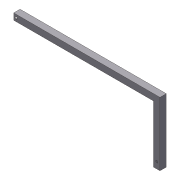
# Autodesk Inventor part: LoweringArm
Saved by Autodesk Inventor 2012 (Build 160160000, 160)
## iProperties
Created: 2012-02-26
Part Number: LoweringArm
Material: Aluminum-6061
Document SubType Name: Modeling
Designer: JesseK
Density: 2.71 g/cm^3
Mass: 259.596 g
Surface Area: 1210.8 cm^2
Volume: 95.7917 cm^3
Author: JesseK
Autodesk Inventor part; units mm, degrees
ref_plane "YZ Plane" through (0, 0, 0) normal (1, 0, 0) x (0, 1, 0)
ref_plane "XZ Plane" through (0, 0, 0) normal (0, 1, 0) x (-1, 0, 0)
ref_plane "XY Plane" through (0, 0, 0) normal (0, 0, 1) x (1, 0, 0)
sketch "Sketch1" plane through (0, 0, 0) normal (0, 0, 1) x (1, 0, 0)
  line L0 (0, 0) -> (-25.4, 0)
  line L1 (-254, 228.6) -> (-254, 254)
  line L2 (-254, 254) -> (0, 254)
  line L3 (0, 254) -> (0, 0)
  line L4 (-25.4, 0) -> (-25.4, 228.6)
  line L5 (-25.4, 228.6) -> (-254, 228.6)
  dimension "d0" = 25.4
  dimension "d1" = 254
  dimension "d2" = 254
  constraints: 12 end point, 2 parallel, 2 perpendicular, 1 horizontal
  measures "d0" distance of L1.start L1.end
  measures "d1" distance of L2.end L0.start
  measures "d2" distance of L1.end L2.end
extrude "Extrusion1" add sketch "Sketch1" along normal blind 25.4
shell "Shell1" thickness 1.5875 removed faces 2 at (-8.4667, 0, 8.4667) at (-254, 237.0667, 8.4667)
sketch "Sketch2" plane through (0, 0, 25.4) normal (0, 0, 1) x (1, 0, 0)
  line L0 (0, 0) -> (-25.4, 0) projected
  line L1 (0, 254) -> (0, 0) projected
  circle A0 centre (-12.7, 25.4) radius 4.7625
  dimension "d6" = 9.525
  dimension "d7" = 12.7
  dimension "d8" = 25.4
  constraints: 1 centre point
  measures "d6" diameter of A0
  measures "d7" distance from line of L1 A0.centre
  measures "d8" distance from line of L0 A0.centre
extrude "Extrusion2" cut sketch "Sketch2" against normal through all
sketch "Sketch3" plane through (0, 0, 0) normal (0, 0, -1) x (-1, 0, 0)
  line L0 (25.4, 228.6) -> (254, 228.6) projected
  line L1 (254, 228.6) -> (254, 254) projected
  circle A0 centre (244.475, 241.3) radius 4.7625
  dimension "d11" = 9.525
  dimension "d12" = 12.7
  dimension "d13" = 9.525
  constraints: 1 centre point
  measures "d11" diameter of A0
  measures "d12" distance from line of L0 A0.centre
  measures "d13" distance from line of L1 A0.centre
extrude "Extrusion3" cut sketch "Sketch3" against normal through all
body "Solid1"
